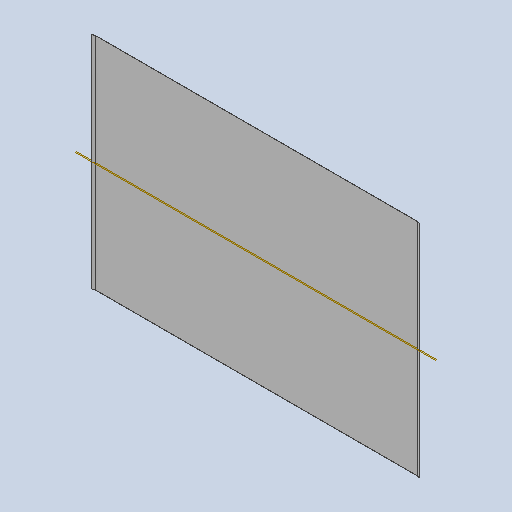
# Autodesk Inventor part: Ke_Bang_Tai
Saved by Autodesk Inventor 2023 (Build 270158000, 158)
## iProperties
Created: 2025-03-29
Part Number: Ke_Bang_Tai
Material: Generic
Document SubType Name: Modeling
Designer: huyqu
Density: 1 g/cm^3
Appearance: Default
Author: huyqu
Autodesk Inventor part; units mm, degrees
ref_plane "YZ Plane" through (0, 0, 0) normal (1, 0, 0) x (0, 1, 0)
ref_plane "XZ Plane" through (0, 0, 0) normal (0, 1, 0) x (-1, 0, 0)
ref_plane "XY Plane" through (0, 0, 0) normal (0, 0, 1) x (1, 0, 0)
sketch "Sketch1" plane through (0, 0, 0) normal (0, 0, 1) x (1, 0, 0)
  line L0 (0, 0) -> (1200, 0)
  line L1 (1200, 0) -> (1200, 820)
  line L2 (1200, 820) -> (0, 820)
  line L3 (0, 820) -> (0, 0)
  dimension "d0" = 820
  dimension "d1" = 1200
  constraints: 8 end point, 2 parallel, 1 horizontal, 1 perpendicular
  measures "d0" distance of L2.end L0.start
  measures "d1" distance of L1.end L2.end
extrude "Extrusion1" add sketch "Sketch1" along normal blind 0.8
sketch "Sketch4" plane through (0, 0, 0) normal (0, -1, 0) x (1, 0, 0)
  line L0 (1200, 0) -> (0, 0) projected
  line L1 (0, 0) -> (-9.3969, 3.4202)
  line L2 (0, 0) -> (0, 0.8) projected
  line L3 (0, 0.8) -> (-9.3969, 4.2202)
  line L4 (-9.3969, 3.4202) -> (-9.3969, 4.2202)
  dimension "d16" = 70
  dimension "d17" = 10
  dimension "d18" = 70
  dimension "d19" = 10
  constraints: 6 end point
  measures "d16" angle of L1 L2
  measures "d17" distance of L0.end L1.end
  measures "d18" angle of L2 L3
  measures "d19" distance of L2.end L3.end
extrude "Extrusion4" add sketch "Sketch4" against normal up to surface (820 mm away)
sketch "Sketch5" plane through (0, 0, 0) normal (0, -1, 0) x (1, 0, 0)
  line L0 (1200, 0) -> (1200, 0.8) projected
  line L1 (1200, 0) -> (1209.3969, 3.4202)
  line L2 (1200, 0.8) -> (1209.3969, 4.2202)
  line L3 (1209.3969, 3.4202) -> (1209.3969, 4.2202)
  point P0 (0, 0)
  dimension "d22" = 70
  dimension "d23" = 10
  dimension "d24" = 70
  dimension "d25" = 10
  constraints: 6 end point
  measures "d22" angle of L0 L1
  measures "d23" distance of L0.start L1.end
  measures "d24" angle of L0 L2
  measures "d25" distance of L0.end L2.end
extrude "Extrusion5" add sketch "Sketch5" against normal up to surface (820 mm away)
sketch "Sketch7" plane through (0, 0, 0.8) normal (0, 0, 1) x (1, 0, 0)
  circle A0 centre (56.6674, 837.4999) radius 7.5 projected
  line L0 (19.1715, 870) -> (19.1715, -50) projected
  circle A1 centre (1126.6715, 837.4999) radius 7.5
  line L1 (1159.1715, 870) -> (1159.1715, -50) projected
  point P0 (0, 0)
  dimension "d30" = 15
  dimension "d31" = 32.5
  constraints: 1 centre point, 1 horizontal alignment
  measures "d30" diameter of A1
  measures "d31" distance from line of L1 A1.centre
extrude "Extrusion6" cut sketch "Sketch7" against normal blind 10
ref_plane "Work Plane2" through (0, 410, 0) normal (0, -1, 0) x (1, 0, 0)
mirror "Mirror2" about plane through (0, 410, 0) normal (0, -1, 0) of "Extrusion6"
body "Solid1"
